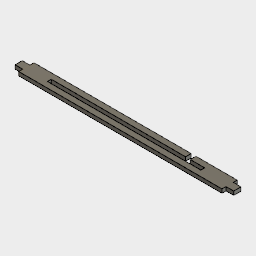
rail (Autodesk Fusion 360 design; units mm, degrees)
Autodesk Fusion 360 part; units mm, degrees
sketch "Sketch1" plane through (0, 0, 0) normal (0, 1, 0) x (1, 0, 0)
  line L0 (0, 0) -> (-265, 0)
  line L1 (-265, 0) -> (-265, -20)
  line L2 (-265, -20) -> (0, -20)
  line L3 (0, -20) -> (0, 0)
  dimension "d1" = 265
  dimension "d2" = 20
  measures "d1" distance of L0.start L0.end
  measures "d2" distance of L0.start L2.end
extrude "Extrude1" add sketch "Sketch1" along normal blind 5
sketch "Sketch3" plane through (0, 0, 0) normal (0, 1, 0) x (1, 0, 0)
  line L0 (-235, -7.5) -> (-35, -7.5)
  line L1 (-35, -7.5) -> (-35, -12.5)
  line L2 (-35, -12.5) -> (-235, -12.5)
  line L3 (-235, -12.5) -> (-235, -7.5)
  line L4 (0, 0) -> (-265, 0)
  line L5 (0, -20) -> (0, 0)
  dimension "d9" = 200
  dimension "d10" = 5
  measures "d9" distance of L0.start L0.end
  measures "d10" distance of L0.start L2.end
extrude "Extrude2" cut sketch "Sketch3" along normal blind 5
sketch "Sketch4" plane through (0, 0, 0) normal (0, 1, 0) x (1, 0, 0)
  line L0 (0, -5.25) -> (5, -5.25)
  line L1 (5, -5.25) -> (5, -14.75)
  line L2 (5, -14.75) -> (0, -14.75)
  line L3 (0, -14.75) -> (0, -5.25)
  line L4 (0, -20) -> (0, 0)
  dimension "d13" = 5
  dimension "d14" = 9.5
  measures "d13" distance of L0.start L0.end
  measures "d14" distance of L0.start L2.end
extrude "Extrude3" add sketch "Sketch4" along normal blind 5
sketch "Sketch5" plane through (-265, 0, 0) normal (-1, 0, 0) x (0, 0, 1)
  line L0 (0, 0) -> (20, 0)
  line L1 (20, 0) -> (20, 5)
  line L2 (20, 5) -> (0, 5)
  line L3 (0, 5) -> (0, 0)
sketch "Sketch6" plane through (0, 0, 0) normal (0, 1, 0) x (1, 0, 0)
  line L0 (-265, -5.25) -> (-270, -5.25)
  line L1 (-270, -5.25) -> (-270, -14.75)
  line L2 (-270, -14.75) -> (-265, -14.75)
  line L3 (-265, -14.75) -> (-265, -5.25)
  line L4 (-265, 0) -> (-265, -20)
  line L5 (-265, -20) -> (-265, 0)
  dimension "d17" = 9.5
  dimension "d18" = 5
  measures "d17" distance of L0.start L2.end
  measures "d18" distance of L0.start L0.end
extrude "Extrude4" add sketch "Sketch6" along normal blind 5
sketch "Sketch7" plane through (0, 0, 0) normal (0, 1, 0) x (1, 0, 0)
  line L0 (-60, 0) -> (-54, 0)
  line L1 (-54, 0) -> (-54, -7.5)
  line L2 (-54, -7.5) -> (-60, -7.5)
  line L3 (-60, -7.5) -> (-60, 0)
  line L4 (0, 0) -> (-265, 0)
  dimension "d21" = 6
  dimension "d22" = 7.5
  measures "d21" distance of L0.start L0.end
  measures "d22" distance of L0.start L2.end
extrude "Extrude5" cut sketch "Sketch7" along normal blind 5
sketch "Sketch8" plane through (0, 0, 0) normal (0, 1, 0) x (1, 0, 0)
  line L0 (5, -5.25) -> (10, -5.25)
  line L1 (10, -5.25) -> (10, -14.75)
  line L2 (10, -14.75) -> (5, -14.75)
  line L3 (5, -14.75) -> (5, -5.25)
  point P0 (5, -5.25)
  dimension "d25" = 9.5
  measures "d25" distance of P0 L2.end
extrude "Extrude6" add sketch "Sketch8" along normal blind 5
sketch "Sketch9" plane through (0, 0, 0) normal (0, 1, 0) x (1, 0, 0)
  line L0 (-270, -5.25) -> (-275, -5.25)
  line L1 (-275, -5.25) -> (-275, -14.75)
  line L2 (-275, -14.75) -> (-270, -14.75)
  line L3 (-270, -14.75) -> (-270, -5.25)
  point P0 (-270, -5.25)
  dimension "d28" = 5
  dimension "d29" = 9.5
  measures "d28" distance of P0 L0.end
  measures "d29" distance of P0 L2.end
extrude "Extrude7" add sketch "Sketch9" along normal blind 5
